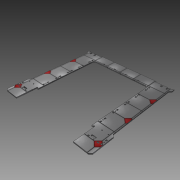
# Autodesk Inventor part: frame
Saved by Autodesk Inventor 2014 (Build 180170000, 170)
## iProperties
Created: 2013-12-06
Part Number: frame
Material: Generic
Document SubType Name: Modeling
Designer: buben
Density: 1 g/cm^3
Appearance: Anodized - Dark Gray
Author: buben
Subject: Laser Cutted
Autodesk Inventor part; units mm, degrees
ref_plane "YZ Plane" through (0, 0, 0) normal (1, 0, 0) x (0, 1, 0)
ref_plane "XZ Plane" through (0, 0, 0) normal (0, 1, 0) x (-1, 0, 0)
ref_plane "XY Plane" through (0, 0, 0) normal (0, 0, 1) x (1, 0, 0)
sketch "Sketch1" plane through (0, 0, 0) normal (0, 0, 1) x (1, 0, 0)
  line L0 (0, 504) -> (509, 504)
  line L1 (0, 10) -> (10, 0)
  line L2 (509, 10) -> (499, 0)
  line L3 (0, 487) -> (10, 477)
  line L4 (10, 477) -> (10, 120)
  line L5 (10, 120) -> (0, 110)
  line L6 (509, 487) -> (499, 477)
  line L7 (499, 477) -> (499, 120)
  line L8 (499, 120) -> (509, 110)
  line L9 (0, 10) -> (0, 110)
  line L10 (0, 487) -> (0, 504)
  line L11 (509, 504) -> (509, 487)
  line L12 (509, 110) -> (509, 10)
  line L13 (10, 0) -> (81, 0)
  line L14 (81, 0) -> (81, 104)
  line L15 (499, 0) -> (428, 0)
  line L16 (428, 0) -> (428, 104)
  line L17 (81, 104) -> (87, 104)
  line L18 (87, 104) -> (87, 100)
  line L19 (87, 100) -> (93, 100)
  line L20 (93, 100) -> (93, 434)
  line L21 (428, 104) -> (422, 104)
  line L22 (422, 104) -> (422, 100)
  line L23 (422, 100) -> (416, 100)
  line L24 (416, 100) -> (416, 434)
  line L25 (93, 434) -> (103, 444)
  line L26 (103, 444) -> (406, 444)
  line L27 (406, 444) -> (416, 434)
  point P0 (0, 0)
  point P1 (254.5, 444)
  point P2 (254.5, 504)
  dimension "d0" = 509
  dimension "d1" = 504
  dimension "d2" = 10
  dimension "d3" = 10
  dimension "d4" = 45
  dimension "d5" = 10
  dimension "d6" = 17
  dimension "d7" = 6
  dimension "d8" = 6
  dimension "d9" = 6
  dimension "d10" = 6
  dimension "d11" = 4
  dimension "d12" = 10
  dimension "d13" = 60
  dimension "d14" = 323
  dimension "d15" = 104
  dimension "d18" = 6
  constraints: 56 end point, 17 perpendicular, 12 parallel, 7 horizontal alignment, 3 vertical alignment, 2 collinear, 2 midpoint, 2 vertical
  measures "d0" distance of L0.start L0.end
  measures "d1" distance from line of L0 L1.end
  measures "d2" distance between parallel lines of L4 L10
  measures "d3" distance between parallel lines of L11 L7
  measures "d4" angle of L1 L13
  measures "d5" horizontal distance of L1.start L1.end
  measures "d6" distance of L3.start L0.start
  measures "d7" distance of L14.end L17.end
  measures "d8" distance of L16.end L21.end
  measures "d9" distance of L18.end L19.end
  measures "d10" distance of L22.end L23.end
  measures "d11" distance of L17.end L18.end
  measures "d12" horizontal distance of L20.end L25.end
  measures "d13" distance between parallel lines of L26 L0
  measures "d14" distance between parallel lines of L24 L20
  measures "d15" distance between parallel lines of L13 L17
  measures "d18" vertical distance of L14.end L5.end
extrude "Extrusion1" add sketch "Sketch1" along normal blind 6
sketch "Sketch2" plane through (0, 0, 6) normal (0, 0, 1) x (1, 0, 0)
  line L0 (103, 444) -> (406, 444) projected
  line L1 (216.2, 456) -> (224.2, 456)
  line L2 (224.2, 456) -> (224.2, 450)
  line L3 (224.2, 450) -> (216.2, 450)
  line L4 (216.2, 450) -> (216.2, 456)
  line L5 (284.8, 456) -> (292.8, 456)
  line L6 (292.8, 456) -> (292.8, 450)
  line L7 (292.8, 450) -> (284.8, 450)
  line L8 (284.8, 450) -> (284.8, 456)
  line L9 (353.4, 456) -> (361.4, 456)
  line L10 (361.4, 456) -> (361.4, 450)
  line L11 (361.4, 450) -> (353.4, 450)
  line L12 (353.4, 450) -> (353.4, 456)
  line L13 (147.6, 456) -> (155.6, 456)
  line L14 (155.6, 456) -> (155.6, 450)
  line L15 (155.6, 450) -> (147.6, 450)
  line L16 (147.6, 450) -> (147.6, 456)
  line L17 (155.6, 453) -> (216.2, 453) construction
  line L18 (224.2, 453) -> (284.8, 453) construction
  line L19 (292.8, 453) -> (353.4, 453) construction
  point P0 (0, 0)
  point P1 (254.5, 453)
  point P2 (254.5, 444)
  dimension "d19" = 8
  dimension "d21" = 6
  dimension "d22" = 60.6
  dimension "d23" = 6
  constraints: 38 end point, 11 collinear, 8 midpoint, 8 parallel, 4 horizontal, 4 perpendicular, 1 vertical alignment
  measures "d19" distance of L13.start L13.end
  measures "d21" distance of L15.end L13.start
  measures "d22" distance of L17.start L17.end
  measures "d23" distance between parallel lines of L0 L3
extrude "Extrusion2" cut sketch "Sketch2" against normal through all
sketch "Sketch3" plane through (0, 0, 6) normal (0, 0, 1) x (1, 0, 0)
  line L0 (509, 504) -> (0, 504) projected
  line L1 (0, 504) -> (0, 487) projected
  line L2 (509, 487) -> (509, 504) projected
  line L3 (6, 504) -> (90, 504)
  line L4 (90, 504) -> (90, 498)
  line L5 (90, 498) -> (6, 498)
  line L6 (6, 498) -> (6, 504)
  line L7 (419, 504) -> (503, 504)
  line L8 (503, 504) -> (503, 498)
  line L9 (503, 498) -> (419, 498)
  line L10 (419, 498) -> (419, 504)
  point P0 (0, 0)
  dimension "d26" = 6
  dimension "d27" = 6
  dimension "d28" = 84
  dimension "d29" = 6
  constraints: 16 end point, 4 parallel, 2 collinear, 2 horizontal, 2 perpendicular, 2 point on line
  measures "d26" distance of L3.end L4.end
  measures "d27" distance between parallel lines of L1 L6
  measures "d28" distance of L4.end L5.end
  measures "d29" distance between parallel lines of L2 L8
extrude "Extrusion3" cut sketch "Sketch3" against normal through all
sketch "Sketch4" plane through (0, 0, 6) normal (0, 0, 1) x (1, 0, 0)
  line L0 (419, 504) -> (90, 504) projected
  line L1 (93, 100) -> (93, 434) projected
  line L2 (103, 444) -> (406, 444) projected
  line L3 (81, 444) -> (87, 444)
  line L4 (87, 444) -> (87, 436)
  line L5 (87, 436) -> (81, 436)
  line L6 (81, 436) -> (81, 444)
  line L7 (81, 421) -> (87, 421)
  line L8 (87, 421) -> (87, 413)
  line L9 (87, 413) -> (81, 413)
  line L10 (81, 413) -> (81, 421)
  line L11 (81, 436) -> (87, 421) construction
  line L12 (81, 421) -> (87, 436) construction
  circle A0 centre (84, 428.5) radius 2.25
  line L13 (81, 374) -> (87, 374)
  line L14 (87, 374) -> (87, 366)
  line L15 (87, 366) -> (81, 366)
  line L16 (81, 366) -> (81, 374)
  line L17 (81, 351) -> (87, 351)
  line L18 (87, 351) -> (87, 343)
  line L19 (87, 343) -> (81, 343)
  line L20 (81, 343) -> (81, 351)
  line L21 (81, 366) -> (87, 351) construction
  line L22 (81, 351) -> (87, 366) construction
  circle A1 centre (84, 358.5) radius 2.25
  line L23 (81, 304) -> (87, 304)
  line L24 (87, 304) -> (87, 296)
  line L25 (87, 296) -> (81, 296)
  line L26 (81, 296) -> (81, 304)
  line L27 (81, 281) -> (87, 281)
  line L28 (87, 281) -> (87, 273)
  line L29 (87, 273) -> (81, 273)
  line L30 (81, 273) -> (81, 281)
  line L31 (81, 296) -> (87, 281) construction
  line L32 (81, 281) -> (87, 296) construction
  circle A2 centre (84, 288.5) radius 2.25
  line L33 (81, 234) -> (87, 234)
  line L34 (87, 234) -> (87, 226)
  line L35 (87, 226) -> (81, 226)
  line L36 (81, 226) -> (81, 234)
  line L37 (81, 211) -> (87, 211)
  line L38 (87, 211) -> (87, 203)
  line L39 (87, 203) -> (81, 203)
  line L40 (81, 203) -> (81, 211)
  line L41 (81, 226) -> (87, 211) construction
  line L42 (81, 211) -> (87, 226) construction
  circle A3 centre (84, 218.5) radius 2.25
  line L43 (81, 164) -> (87, 164)
  line L44 (87, 164) -> (87, 156)
  line L45 (87, 156) -> (81, 156)
  line L46 (81, 156) -> (81, 164)
  line L47 (81, 141) -> (87, 141)
  line L48 (87, 141) -> (87, 133)
  line L49 (87, 133) -> (81, 133)
  line L50 (81, 133) -> (81, 141)
  line L51 (81, 156) -> (87, 141) construction
  line L52 (81, 141) -> (87, 156) construction
  circle A4 centre (84, 148.5) radius 2.25
  line L53 (254.5, 504) -> (254.5, 444) construction
  line L54 (428, 444) -> (422, 444)
  line L55 (422, 444) -> (422, 436)
  line L56 (422, 436) -> (428, 436)
  line L57 (428, 436) -> (428, 444)
  line L58 (428, 421) -> (422, 421)
  line L59 (422, 421) -> (422, 413)
  line L60 (422, 413) -> (428, 413)
  line L61 (428, 413) -> (428, 421)
  line L62 (428, 436) -> (422, 421) construction
  line L63 (428, 421) -> (422, 436) construction
  circle A5 centre (425, 428.5) radius 2.25
  line L64 (428, 374) -> (422, 374)
  line L65 (422, 366) -> (428, 366)
  line L66 (428, 366) -> (428, 374)
  line L67 (422, 374) -> (422, 366)
  circle A6 centre (425, 358.5) radius 2.25
  line L68 (428, 351) -> (422, 351)
  line L69 (428, 366) -> (422, 351) construction
  line L70 (428, 351) -> (422, 366) construction
  line L71 (428, 343) -> (428, 351)
  line L72 (422, 343) -> (428, 343)
  line L73 (422, 351) -> (422, 343)
  line L74 (428, 304) -> (422, 304)
  line L75 (422, 296) -> (428, 296)
  line L76 (428, 296) -> (428, 304)
  line L77 (422, 304) -> (422, 296)
  circle A7 centre (425, 288.5) radius 2.25
  line L78 (428, 281) -> (422, 281)
  line L79 (428, 296) -> (422, 281) construction
  line L80 (428, 281) -> (422, 296) construction
  line L81 (428, 273) -> (428, 281)
  line L82 (422, 273) -> (428, 273)
  line L83 (422, 281) -> (422, 273)
  line L84 (428, 234) -> (422, 234)
  line L85 (422, 226) -> (428, 226)
  line L86 (428, 226) -> (428, 234)
  line L87 (422, 234) -> (422, 226)
  circle A8 centre (425, 218.5) radius 2.25
  line L88 (428, 211) -> (422, 211)
  line L89 (428, 226) -> (422, 211) construction
  line L90 (428, 211) -> (422, 226) construction
  line L91 (428, 203) -> (428, 211)
  line L92 (422, 203) -> (428, 203)
  line L93 (422, 211) -> (422, 203)
  line L94 (428, 164) -> (422, 164)
  line L95 (422, 156) -> (428, 156)
  line L96 (428, 156) -> (428, 164)
  line L97 (422, 164) -> (422, 156)
  circle A9 centre (425, 148.5) radius 2.25
  line L98 (428, 141) -> (422, 141)
  line L99 (428, 156) -> (422, 141) construction
  line L100 (428, 141) -> (422, 156) construction
  line L101 (428, 133) -> (428, 141)
  line L102 (422, 133) -> (428, 133)
  line L103 (422, 141) -> (422, 133)
  point P0 (0, 0)
  dimension "d32" = 8
  dimension "d33" = 8
  dimension "d34" = 6
  dimension "d35" = 15
  dimension "d36" = 4.5
  dimension "d37" = 6
  dimension "d40" = 70
  constraints: 202 end point, 45 symmetric about line, 10 centre point, 4 parallel, 3 collinear, 3 midpoint, 2 horizontal, 2 perpendicular, 1 vertical, 85 other
  measures "d32" distance of L5.end L3.start
  measures "d33" distance of L9.end L7.start
  measures "d34" distance of L3.start L3.end
  measures "d35" distance between parallel lines of L7 L5
  measures "d36" diameter of A0
  measures "d37" distance between parallel lines of L1 L4
  measures "d40" distance of L3.end L13.end
extrude "Extrusion4" cut sketch "Sketch4" against normal through all
sketch "Sketch7" plane through (0, 0, 6) normal (0, 0, 1) x (1, 0, 0)
  line L0 (422, 304) -> (428, 304) projected
  line L1 (419, 504) -> (90, 504) projected
  line L2 (0, 110) -> (0, 10) projected
  line L3 (10, 0) -> (81, 0) projected
  line L4 (103, 444) -> (406, 444) projected
  line L5 (254.5, 504) -> (254.5, 444) construction
  line L6 (41.5, 64) -> (56.5, 64) construction
  line L7 (41.5, 60) -> (56.5, 60)
  line L8 (56.5, 68) -> (41.5, 68)
  arc A0 (41.5, 68) -> (41.5, 60) centre (41.5, 64) ccw
  arc A1 (56.5, 60) -> (56.5, 68) centre (56.5, 64) ccw
  line L9 (467.5, 64) -> (452.5, 64) construction
  line L10 (467.5, 60) -> (452.5, 60)
  line L11 (452.5, 68) -> (467.5, 68)
  arc A2 (467.5, 60) -> (467.5, 68) centre (467.5, 64) ccw
  arc A3 (452.5, 68) -> (452.5, 60) centre (452.5, 64) ccw
  point P0 (0, 0)
  point P1 (49, 64)
  point P2 (460, 64)
  dimension "d59" = 15
  dimension "d60" = 8
  dimension "d61" = 49
  dimension "d62" = 64
  constraints: 18 end point, 8 point on circle, 7 symmetric about line, 4 centre point, 4 tangent, 3 midpoint, 2 parallel, 2 other
  measures "d59" distance of L6.start L6.end
  measures "d60" distance between parallel lines of L7 L8
  measures "d61" distance from line of L2 point (49, 64)
  measures "d62" distance between parallel lines of L3 L6
extrude "Extrusion7" cut sketch "Sketch7" against normal blind 6
sketch "Sketch8" plane through (0, 0, 6) normal (0, 0, 1) x (1, 0, 0)
  line L0 (56.5, 60) -> (41.5, 60) projected
  line L1 (419, 504) -> (90, 504) projected
  line L2 (0, 110) -> (0, 10) projected
  line L3 (81, 0) -> (81, 104) projected
  line L4 (103, 444) -> (406, 444) projected
  line L5 (16, 58) -> (24, 58)
  line L6 (24, 58) -> (24, 52)
  line L7 (24, 52) -> (16, 52)
  line L8 (16, 52) -> (16, 58)
  line L9 (61, 58) -> (69, 58)
  line L10 (69, 58) -> (69, 52)
  line L11 (69, 52) -> (61, 52)
  line L12 (61, 52) -> (61, 58)
  circle A0 centre (40.5, 55) radius 2.25
  line L13 (254.5, 504) -> (254.5, 444) construction
  line L14 (493, 58) -> (485, 58)
  line L15 (485, 58) -> (485, 52)
  line L16 (485, 52) -> (493, 52)
  line L17 (493, 52) -> (493, 58)
  line L18 (448, 58) -> (440, 58)
  line L19 (440, 58) -> (440, 52)
  line L20 (440, 52) -> (448, 52)
  line L21 (448, 52) -> (448, 58)
  circle A1 centre (468.5, 55) radius 2.25
  point P0 (0, 0)
  point P1 (24, 55)
  point P2 (485, 55)
  dimension "d65" = 8
  dimension "d66" = 8
  dimension "d67" = 6
  dimension "d68" = 4.5
  dimension "d69" = 2
  dimension "d70" = 12
  dimension "d71" = 16
  dimension "d72" = 40.5
  constraints: 34 end point, 10 symmetric about line, 4 parallel, 3 midpoint, 2 centre point, 2 collinear, 2 horizontal, 2 perpendicular, 1 horizontal alignment, 1 other
  measures "d65" distance of L5.start L5.end
  measures "d66" distance of L9.start L9.end
  measures "d67" distance of L7.end L5.start
  measures "d68" diameter of A0
  measures "d69" distance between parallel lines of L5 L0
  measures "d70" distance between parallel lines of L3 L10
  measures "d71" distance between parallel lines of L2 L8
  measures "d72" distance from line of L3 A0.centre
extrude "Extrusion8" cut sketch "Sketch8" against normal blind 6
sketch "Sketch9" plane through (0, 0, 6) normal (0, 0, 1) x (1, 0, 0)
  line L0 (419, 504) -> (90, 504) projected
  line L1 (0, 110) -> (0, 10) projected
  line L2 (103, 444) -> (406, 444) projected
  circle A0 centre (20, 107) radius 2.25
  circle A1 centre (50, 107) radius 2.25
  line L3 (254.5, 504) -> (254.5, 444) construction
  circle A2 centre (489, 107) radius 2.25
  circle A3 centre (459, 107) radius 2.25
  point P0 (0, 0)
  dimension "d75" = 4.5
  dimension "d76" = 30
  dimension "d77" = 20
  dimension "d78" = 3
  constraints: 4 centre point, 2 end point, 2 midpoint, 2 symmetric about line, 1 equal radius, 1 horizontal alignment, 2 other
  measures "d75" diameter of A0
  measures "d76" distance of A1.centre A0.centre
  measures "d77" distance from line of L1 A0.centre
  measures "d78" vertical distance of L1.start A0.centre
extrude "Extrusion9" cut sketch "Sketch9" against normal blind 6
sketch "Sketch10" plane through (0, 0, 6) normal (0, 0, 1) x (1, 0, 0)
  line L0 (419, 504) -> (90, 504) projected
  line L1 (0, 110) -> (0, 10) projected
  line L2 (10, 0) -> (81, 0) projected
  line L3 (103, 444) -> (406, 444) projected
  line L4 (3, 85) -> (9, 85)
  line L5 (9, 85) -> (9, 77)
  line L6 (9, 77) -> (3, 77)
  line L7 (3, 77) -> (3, 85)
  line L8 (3, 62) -> (9, 62)
  line L9 (9, 62) -> (9, 54)
  line L10 (9, 54) -> (3, 54)
  line L11 (3, 54) -> (3, 62)
  line L12 (3, 77) -> (9, 62) construction
  line L13 (3, 62) -> (9, 77) construction
  circle A0 centre (6, 69.5) radius 2.25
  line L14 (254.5, 504) -> (254.5, 444) construction
  line L15 (506, 85) -> (500, 85)
  line L16 (500, 85) -> (500, 77)
  line L17 (500, 77) -> (506, 77)
  line L18 (506, 77) -> (506, 85)
  line L19 (506, 62) -> (500, 62)
  line L20 (500, 62) -> (500, 54)
  line L21 (500, 54) -> (506, 54)
  line L22 (506, 54) -> (506, 62)
  line L23 (506, 77) -> (500, 62) construction
  line L24 (506, 62) -> (500, 77) construction
  circle A1 centre (503, 69.5) radius 2.25
  point P0 (0, 0)
  dimension "d81" = 8
  dimension "d82" = 6
  dimension "d83" = 8
  dimension "d84" = 15
  dimension "d85" = 4.5
  dimension "d86" = 3
  dimension "d87" = 69.5
  constraints: 42 end point, 9 symmetric about line, 4 parallel, 3 midpoint, 2 centre point, 2 collinear, 2 horizontal, 2 perpendicular, 1 other
  measures "d81" distance of L6.end L4.start
  measures "d82" distance of L4.start L4.end
  measures "d83" distance of L10.end L8.start
  measures "d84" distance between parallel lines of L8 L6
  measures "d85" diameter of A0
  measures "d86" distance between parallel lines of L1 L7
  measures "d87" distance from line of L2 A0.centre
extrude "Extrusion10" cut sketch "Sketch10" against normal blind 6
sketch "Sketch14" plane through (0, 0, 6) normal (0, 0, 1) x (1, 0, 0)
  line L0 (419, 504) -> (90, 504) projected
  line L1 (90, 498) -> (6, 498) projected
  line L2 (0, 504) -> (0, 487) projected
  line L3 (103, 444) -> (406, 444) projected
  line L4 (22.75, 498) -> (27.25, 498)
  line L5 (27.25, 481.7) -> (22.75, 481.7)
  line L6 (29.75, 493) -> (29.75, 485.7)
  line L7 (20.25, 485.7) -> (20.25, 493)
  line L8 (20.25, 493) -> (22.75, 493)
  line L9 (27.25, 493) -> (29.75, 493)
  line L10 (29.75, 485.7) -> (27.25, 485.7)
  line L11 (22.75, 485.7) -> (20.25, 485.7)
  line L12 (22.75, 481.7) -> (22.75, 485.7)
  line L13 (22.75, 493) -> (22.75, 498)
  line L14 (27.25, 498) -> (27.25, 493)
  line L15 (27.25, 485.7) -> (27.25, 481.7)
  line L16 (50.301, 498) -> (54.801, 498)
  line L17 (54.801, 481.7) -> (50.301, 481.7)
  line L18 (57.301, 493) -> (57.301, 485.7)
  line L19 (47.801, 485.7) -> (47.801, 493)
  line L20 (47.801, 493) -> (50.301, 493)
  line L21 (54.801, 493) -> (57.301, 493)
  line L22 (57.301, 485.7) -> (54.801, 485.7)
  line L23 (50.301, 485.7) -> (47.801, 485.7)
  line L24 (50.301, 481.7) -> (50.301, 485.7)
  line L25 (50.301, 493) -> (50.301, 498)
  line L26 (54.801, 498) -> (54.801, 493)
  line L27 (54.801, 485.7) -> (54.801, 481.7)
  line L28 (254.5, 504) -> (254.5, 444) construction
  line L29 (486.25, 498) -> (481.75, 498)
  line L30 (481.75, 481.7) -> (486.25, 481.7)
  line L31 (479.25, 493) -> (479.25, 485.7)
  line L32 (488.75, 485.7) -> (488.75, 493)
  line L33 (488.75, 493) -> (486.25, 493)
  line L34 (481.75, 493) -> (479.25, 493)
  line L35 (479.25, 485.7) -> (481.75, 485.7)
  line L36 (486.25, 485.7) -> (488.75, 485.7)
  line L37 (486.25, 481.7) -> (486.25, 485.7)
  line L38 (486.25, 493) -> (486.25, 498)
  line L39 (481.75, 498) -> (481.75, 493)
  line L40 (481.75, 485.7) -> (481.75, 481.7)
  line L41 (451.699, 493) -> (451.699, 485.7)
  line L42 (451.699, 485.7) -> (454.199, 485.7)
  line L43 (454.199, 493) -> (451.699, 493)
  line L44 (454.199, 485.7) -> (454.199, 481.7)
  line L45 (454.199, 498) -> (454.199, 493)
  line L46 (458.699, 481.7) -> (458.699, 485.7)
  line L47 (454.199, 481.7) -> (458.699, 481.7)
  line L48 (458.699, 493) -> (458.699, 498)
  line L49 (458.699, 498) -> (454.199, 498)
  line L50 (458.699, 485.7) -> (461.199, 485.7)
  line L51 (461.199, 485.7) -> (461.199, 493)
  line L52 (461.199, 493) -> (458.699, 493)
  point P0 (0, 0)
  point P1 (25, 481.7)
  point P2 (52.551, 481.7)
  point P3 (484, 481.7)
  point P4 (456.449, 481.7)
  dimension "d124" = 4.5
  dimension "d125" = 4
  dimension "d126" = 5
  dimension "d127" = 7.3
  dimension "d128" = 2.5
  dimension "d129" = 4.5
  dimension "d130" = 4
  dimension "d131" = 5
  dimension "d132" = 7.3
  dimension "d133" = 2.5
  dimension "d134" = 52.551
  dimension "d135" = 25
  constraints: 98 end point, 26 symmetric about line, 20 parallel, 12 collinear, 8 perpendicular, 6 horizontal, 4 midpoint
  measures "d124" distance of L5.start L5.end
  measures "d125" distance of L5.end L11.start
  measures "d126" distance of L8.end L4.start
  measures "d127" distance of L7.start L7.end
  measures "d128" distance of L7.end L8.end
  measures "d129" distance of L27.end L24.start
  measures "d130" distance of L24.start L24.end
  measures "d131" distance of L25.start L25.end
  measures "d132" distance of L23.end L19.end
  measures "d133" distance of L19.end L25.start
  measures "d134" distance from line of point (52.551, 481.7) L2
  measures "d135" distance from line of L2 point (25, 481.7)
extrude "Extrusion14" cut sketch "Sketch14" against normal through all
equation "\"d3\" = d2"
equation "\"d8\" = d7"
equation "\"d9\" = d7"
equation "\"d10\" = d8"
body "Solid1"
